Autodesk Inventor part; units mm, degrees
(part 3 of 3)
  spline S454 degree 2 poles (77.0165, -133.4993) (77.0455, -133.396) (77.1198, -133.396) knots 0 0 0 1 1 1
  spline S455 degree 2 poles (77.1198, -133.396) (77.1942, -133.396) (77.2204, -133.4663) knots 0 0 0 1 1 1
  line L300 (77.2204, -133.4663) -> (77.6983, -134.7693)
  spline S456 degree 2 poles (77.6983, -134.7693) (77.7039, -134.7831) (77.7039, -134.7996) knots 0 0 0 1 1 1
  spline S457 degree 2 poles (77.2796, -133.1494) (77.2218, -133.1494) (77.1639, -133.1205) knots 0 0 0 1 1 1
  spline S458 degree 2 poles (77.1639, -133.1205) (77.1047, -133.0861) (77.073, -133.0682) knots 0 0 0 1 1 1
  spline S459 degree 2 poles (77.073, -133.0682) (77.0482, -133.0585) (77.0028, -133.0255) knots 0 0 0 1 1 1
  spline S460 degree 2 poles (77.0028, -133.0255) (76.9738, -133.0048) (76.9601, -133.0048) knots 0 0 0 1 1 1
  spline S461 degree 2 poles (76.9601, -133.0048) (76.9353, -133.0048) (76.8402, -133.0764) (76.8003, -133.0764) knots 0 0 0 1 2 2 2
  spline S462 degree 2 poles (76.8003, -133.0764) (76.759, -133.0764) (76.6956, -133.02) (76.6956, -132.9814) knots 0 0 0 1 2 2 2
  spline S463 degree 2 poles (76.6956, -132.9814) (76.6956, -132.9332) (76.7755, -132.8988) knots 0 0 0 1 1 1
  spline S464 degree 2 poles (76.7755, -132.8988) (76.8168, -132.8519) (76.8485, -132.8368) knots 0 0 0 1 1 1
  spline S465 degree 2 poles (76.8485, -132.8368) (76.8939, -132.8134) (76.9601, -132.8134) knots 0 0 0 1 1 1
  spline S466 degree 2 poles (76.9601, -132.8134) (77.0124, -132.8134) (77.073, -132.8423) knots 0 0 0 1 1 1
  spline S467 degree 2 poles (77.073, -132.8423) (77.1157, -132.8657) (77.157, -132.8891) knots 0 0 0 1 1 1
  spline S468 degree 2 poles (77.157, -132.8891) (77.1846, -132.9001) (77.2342, -132.936) knots 0 0 0 1 1 1
  spline S469 degree 2 poles (77.2342, -132.936) (77.2658, -132.9594) (77.2796, -132.9594) knots 0 0 0 1 1 1
  spline S470 degree 2 poles (77.2796, -132.9594) (77.3044, -132.9594) (77.4008, -132.8864) (77.4394, -132.8864) knots 0 0 0 1 2 2 2
  spline S471 degree 2 poles (77.4394, -132.8864) (77.5427, -132.8864) (77.5427, -132.9814) knots 0 0 0 1 1 1
  spline S472 degree 2 poles (77.5427, -132.9814) (77.5427, -133.0255) (77.5, -133.0599) knots 0 0 0 1 1 1
  spline S473 degree 2 poles (77.5, -133.0599) (77.4683, -133.0806) (77.4366, -133.1026) knots 0 0 0 1 1 1
  spline S474 degree 2 poles (77.4366, -133.1026) (77.3664, -133.1494) (77.2796, -133.1494) knots 0 0 0 1 1 1
  line L301 (77.1198, -133.7445) -> (76.9077, -134.3409)
  line L302 (76.9077, -134.3409) -> (77.332, -134.3409)
  line L303 (77.332, -134.3409) -> (77.1198, -133.7445)
  spline S475 degree 2 poles (79.0152, -134.436) (79.0152, -134.6274) (78.719, -134.896) (78.511, -134.896) knots 0 0 0 1 2 2 2
  spline S476 degree 2 poles (78.511, -134.896) (78.3017, -134.896) (78.0069, -134.6274) (78.0069, -134.436) knots 0 0 0 1 2 2 2
  line L304 (78.0069, -134.436) -> (78.0069, -133.8533)
  spline S477 degree 2 poles (78.0069, -133.8533) (78.0069, -133.6632) (78.3017, -133.3946) (78.511, -133.3946) knots 0 0 0 1 2 2 2
  spline S478 degree 2 poles (78.511, -133.3946) (78.7204, -133.3946) (79.0152, -133.6618) (79.0152, -133.8533) knots 0 0 0 1 2 2 2
  line L305 (79.0152, -133.8533) -> (79.0152, -134.436)
  line L306 (78.8085, -134.436) -> (78.8085, -133.8533)
  spline S479 degree 2 poles (78.8085, -133.8533) (78.8085, -133.7417) (78.6364, -133.5861) (78.511, -133.5861) knots 0 0 0 1 2 2 2
  spline S480 degree 2 poles (78.511, -133.5861) (78.3857, -133.5861) (78.2135, -133.7417) (78.2135, -133.8533) knots 0 0 0 1 2 2 2
  line L307 (78.2135, -133.8533) -> (78.2135, -134.436)
  spline S481 degree 2 poles (78.2135, -134.436) (78.2135, -134.5489) (78.3857, -134.7045) (78.511, -134.7045) knots 0 0 0 1 2 2 2
  spline S482 degree 2 poles (78.511, -134.7045) (78.6364, -134.7045) (78.8085, -134.5489) (78.8085, -134.436) knots 0 0 0 1 2 2 2
  point P0 (0, 0)
  point P1 (-20, -105)
  point P2 (0, -120)
  point P3 (20, -105)
  point P4 (-20, -132)
  point P5 (-120, -132)
  point P6 (-70, -128.5)
  point P7 (85, -130.5)
  point P8 (85, -134)
  point P9 (50.965, -135.4999)
  dimension "d93" = 8.07
  dimension "d95" = 6.9999
  dimension "d67" = 35
  dimension "d68" = 40
  dimension "d69" = 15
  dimension "d70" = 0.1
  dimension "d71" = 1
  dimension "d72" = 0.9
  dimension "d87" = 7
  dimension "d88" = 100
  dimension "d89" = 30
  dimension "d90" = 2
  dimension "d91" = 3
  dimension "d92" = 6
  dimension "d94" = 4.035
  dimension "d96" = 0.4999
  dimension "d97" = 70
  dimension "d98" = 8
  dimension "d99" = 70
  constraints: 14 end point, 12 point on circle, 12 tangent, 8 point on line, 7 midpoint, 6 centre point, 4 equal radius, 2 horizontal, 2 parallel, 1 collinear, 1 perpendicular, 1 symmetric about line, 10 other
  measures "d67" distance between parallel lines of L5 L4
  measures "d68" distance of point (-20, -105) point (20, -105)
  measures "d69" distance from line of L4 point (0, -120)
  measures "d70" distance between parallel lines of L2 L6
  measures "d71" radius of A0
  measures "d72" radius of A3
  measures "d87" distance between parallel lines of L12 L11
  measures "d88" distance of L10.end L11.end
  measures "d89" distance from line of point (85, -130.5) L13
  measures "d90" distance of L19.end L20.end
  measures "d91" distance of L14.end L15.end
  measures "d92" distance between parallel lines of L14 L19
  measures "d94" distance from line of L13 point (50.965, -135.5)
  measures "d97" distance from line of L1 point (-70, -128.5)
  measures "d98" distance from line of L5 point (-120, -132)
  measures "d99" distance between parallel lines of L1 L18
emboss "Relevo1" sketch "Esboço6" operation cut depth 0.1 direction (0, 0, -1)
equation "\"d94\" = 0.5 * d93"
equation "\"d85\" = d86"
equation "\"d72\" = d71 - d70"
equation "\"d96\" = -0.5 * d92 + 0.5 * d95"
